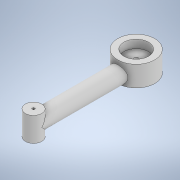
# Autodesk Inventor part: Intermediate Link 2
Saved by Autodesk Inventor 2020 (Build 240168000, 168)
## iProperties
Created: 2022-02-15
Part Number: Intermediate Link 2
Material: Generic
Document SubType Name: Modeling
Designer: New-Computer
Density: 1 g/cm^3
Appearance: Default
Mass: 2187.16 g
Surface Area: 1296.73 cm^2
Volume: 2187.16 cm^3
Author: New-Computer
Autodesk Inventor part; units mm, degrees
ref_plane "YZ Plane" through (0, 0, 0) normal (1, 0, 0) x (0, 1, 0)
ref_plane "XZ Plane" through (0, 0, 0) normal (0, 1, 0) x (-1, 0, 0)
ref_plane "XY Plane" through (0, 0, 0) normal (0, 0, 1) x (1, 0, 0)
sketch "Sketch1" plane through (0, 0, 0) normal (0, 0, 1) x (1, 0, 0)
  circle A0 centre (0, 0) radius 20
  dimension "d0" = 40
  constraints: 1 centre point, 1 coincident
  measures "d0" diameter of A0
extrude "Extrusion1" add sketch "Sketch1" along normal blind 250
sketch "Sketch2" plane through (0, 0, 0) normal (0, 1, 0) x (-1, 0, 0)
  line L0 (20, 0) -> (-20, 0) projected
  circle A0 centre (0, 0) radius 45
  dimension "d3" = 90
  constraints: 1 centre point, 1 coincident
  measures "d3" diameter of A0
extrude "Extrusion2" add sketch "Sketch2" along normal blind 30 and the other way blind 20
sketch "Sketch4" plane through (0, 30, 0) normal (0, 1, 0) x (1, 0, 0)
  circle A0 centre (0, 0) radius 5
  dimension "d9" = 10
  constraints: 1 centre point, 1 coincident
  measures "d9" diameter of A0
extrude "Extrusion4" cut sketch "Sketch4" along normal through all both and the other way through all
sketch "Sketch6" plane through (0, 30, 0) normal (0, 1, 0) x (1, 0, 0)
  circle A0 centre (0, 0) radius 5 projected
  circle A1 centre (0, 0) radius 30
  circle A2 centre (0, 0) radius 15
  dimension "d15" = 60
  dimension "d16" = 30
  constraints: 2 centre point, 2 coincident
  measures "d15" diameter of A1
  measures "d16" diameter of A2
extrude "Extrusion6" cut sketch "Sketch6" against normal blind 20 contours A1 | A2
sketch "Sketch10" plane through (0, 0, 0) normal (0, 1, 0) x (-1, 0, 0)
  line L0 (20, 250) -> (-20, 250) projected
  circle A0 centre (0, 250) radius 20
  point P0 (0, 0)
  constraints: 1 coincident, 1 horizontal alignment, 1 midpoint, 2 other
extrude "Extrusion8" add sketch "Sketch10" along normal mid plane 59
sketch "Sketch11" plane through (0, 29.5, 250) normal (0, 1, 0) x (1, 0, 0)
  circle A0 centre (0, 0) radius 20 projected
  arc A1 (20, 0) -> (-20, 0) centre (0, 0) ccw projected
  line L0 (-2.5, 2.5) -> (2.5, 2.5)
  line L1 (2.5, 2.5) -> (2.5, -2.5)
  line L2 (2.5, -2.5) -> (-2.5, -2.5)
  line L3 (-2.5, -2.5) -> (-2.5, 2.5)
  line L4 (-2.5, 2.5) -> (2.5, -2.5) construction
  line L5 (2.5, 2.5) -> (-2.5, -2.5) construction
  point P0 (0, 250)
  dimension "d54" = 5
  constraints: 12 end point, 2 midpoint, 2 parallel, 2 perpendicular, 1 coincident, 1 horizontal
  measures "d54" distance of L0.start L0.end
extrude "Extrusion9" cut sketch "Sketch11" against normal through all contours L0 L1 L2 L3
sketch "Sketch12" plane through (0, -20, 0) normal (0, -1, 0) x (1, 0, 0)
  point P0 (0, 0)
sketch "Sketch13" plane through (0, -20, 0) normal (0, -1, 0) x (1, 0, 0)
  point P0 (0, 0)
  point P1 (0, 0)
  point P2 (37.5, 0)
  dimension "d57" = 37.5
  measures "d57" distance of point (0, 0) point (37.5, 0)
hole "Hole3" at (37.5, -20, 0) direction (0, 1, 0) diameter 6 depth 30 tip angle 118
thread "Thread3" size "M6x1" class "6H" standard "ANSI Metric M Profile" length 25
pattern_circular "Circular Pattern3" count 6 over 360 about axis through (0, 30, 0) along (0, 1, 0) of "Hole3"
body "Solid1"
